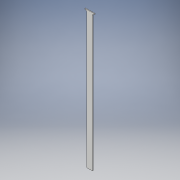
# Autodesk Inventor part: Fuehrungsschiene
Saved by Autodesk Inventor 2017 (Build 210142000, 142)
## iProperties
Part Number: Fuehrungsschiene
Material: Generisch
Document SubType Name: Modeling
Designer: Julian
Density: 1 g/cm^3
Appearance: Vorgabe
Author: Julian
Autodesk Inventor part; units mm, degrees
ref_plane "YZ Plane" through (0, 0, 0) normal (1, 0, 0) x (0, 1, 0)
ref_plane "XZ Plane" through (0, 0, 0) normal (0, 1, 0) x (-1, 0, 0)
ref_plane "XY Plane" through (0, 0, 0) normal (0, 0, 1) x (1, 0, 0)
sketch "Skizze1" plane through (0, 0, 0) normal (0, 1, 0) x (-1, 0, 0)
  line L0 (0, 0) -> (30, 0)
  line L1 (30, 0) -> (30, -1000)
  line L2 (30, -1000) -> (0, -1000)
  line L3 (0, -1000) -> (0, 0)
  line L4 (0, 0) -> (-20, 0)
  line L5 (-5, -20) -> (0, -20)
  arc A0 (0, -20) -> (-20, 0) centre (-20, -20) ccw
  line L6 (30, 0) -> (30, -20)
  line L7 (30, -20) -> (35, -20)
  arc A1 (50, 0) -> (30, -20) centre (50, -20) ccw
  line L8 (50, 0) -> (50, -5)
  arc A2 (50, -5) -> (35, -20) centre (50, -20) ccw
  line L9 (0, -20) -> (-5, -20)
  arc A3 (-5, -20) -> (-20, -5) centre (-20, -20) ccw
  line L10 (35, -20) -> (35, -1000)
  line L11 (35, -1000) -> (30, -1000)
  line L12 (0, -1000) -> (-5, -1000)
  line L13 (-5, -1000) -> (-5, -20)
  line L14 (30, 0) -> (50, 0)
  line L15 (-20, -5) -> (-20, 0)
  line L16 (-20, 0) -> (0, 0)
  line L17 (0, 0) -> (0, -20)
  dimension "d0" = 30
  dimension "d1" = 1000
  dimension "d2" = 20
  dimension "d5" = 20
  dimension "d10" = 5
  dimension "d11" = 5
  dimension "d12" = 5
  constraints: 36 end point, 8 perpendicular, 8 point on circle, 5 point on line, 4 centre point, 3 horizontal, 2 coincident, 2 collinear, 2 vertical, 1 tangent
  measures "d0" distance of L0.start L0.end
  measures "d1" distance of L0.end L1.end
  measures "d2" distance of L0.start L4.end
  measures "d5" distance of L0.end L6.end
  measures "d10" distance of L8.start L8.end
  measures "d11" distance of L5.start L9.start
  measures "d12" distance of L2.end L12.end
extrude "Extrusion1" add sketch "Skizze1" along normal blind 5
